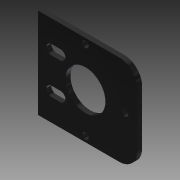
# Autodesk Inventor part: 30288-01
Saved by Autodesk Inventor 2014 (Build 180170000, 170)
## iProperties
Category: NS
Created: 2013-07-17
Part Number: 30288-01
Material: Steel, Mild
Document SubType Name: Modeling
Designer: Edward
Density: 7.86 g/cm^3
Appearance: Lacquer - Black
Description: z-axis motor mount plate (12ga)
Project: Shapeoko
User Status: F
Vendor: ProkTech
Stock Number: SMZM-01
Authority: PER BARRY PROCK 9-16-13 - QUOTE FOR S2ZM-01
Author: Edward
Subject: Structural
Comments: Fusion
Autodesk Inventor part; units mm, degrees
ref_plane "YZ Plane" through (0, 0, 0) normal (1, 0, 0) x (0, 1, 0)
ref_plane "XZ Plane" through (0, 0, 0) normal (0, 1, 0) x (-1, 0, 0)
ref_plane "XY Plane" through (0, 0, 0) normal (0, 0, 1) x (1, 0, 0)
sketch "Sketch1" plane through (0, 0, 0) normal (0, 0, 1) x (1, 0, 0)
  line L0 (-10, -25) -> (45, -25)
  line L1 (45, -25) -> (45, 25)
  line L2 (45, 25) -> (-10, 25)
  line L3 (-10, 25) -> (-10, -25)
  circle A0 centre (16.35, 0) radius 11
  circle A1 centre (38.2703, 0) radius 1.75
  circle A2 centre (16.35, 21.9203) radius 1.75
  circle A3 centre (-5.5703, 0) radius 1.75
  circle A4 centre (16.35, -21.9203) radius 1.75
  line L4 (-2.5, -10) -> (2.5, -10) construction
  line L5 (-2.5, -12.75) -> (2.5, -12.75)
  line L6 (2.5, -7.25) -> (-2.5, -7.25)
  arc A5 (-2.5, -7.25) -> (-2.5, -12.75) centre (-2.5, -10) ccw
  arc A6 (2.5, -12.75) -> (2.5, -7.25) centre (2.5, -10) ccw
  line L7 (-2.5, 7.25) -> (2.5, 7.25)
  line L8 (2.5, 12.75) -> (-2.5, 12.75)
  arc A7 (-2.5, 12.75) -> (-2.5, 7.25) centre (-2.5, 10) ccw
  arc A8 (2.5, 7.25) -> (2.5, 12.75) centre (2.5, 10) ccw
  point P0 (0, 0)
  point P1 (45, 25)
  point P2 (-10, 25)
  point P3 (45, 25)
  point P4 (0, -10)
  dimension "d15" = 0
  dimension "d1" = 22
  dimension "d2" = 25
  dimension "d3" = 26.35
  dimension "d4" = 55
  dimension "d5" = 25
  dimension "d6" = 3.5
  dimension "d7" = 21.9203
  dimension "d8" = 0
  dimension "d11" = 360
  dimension "d13" = 50
  dimension "d14" = 10
  dimension "d16" = 5
  dimension "d17" = 5.5
  dimension "d18" = 10
  dimension "d19" = 15
  dimension "d22" = 20
  constraints: 20 end point, 9 centre point, 8 point on circle, 6 point on line, 5 horizontal, 5 vertical, 4 parallel, 4 tangent, 1 midpoint, 1 perpendicular, 35 other
  measures "d1" diameter of A0
  measures "d2" distance from line of L0 A0.centre
  measures "d3" distance from line of L3 A0.centre
  measures "d4" distance of point (45, 25) point (-10, 25)
  measures "d5" distance from line of point (0, 0) L0
  measures "d6" diameter of A1
  measures "d7" distance of A1.centre A0.centre
  measures "d8" vertical distance of A1.centre A0.centre
  measures "d13" distance of point (45, -25) point (45, 25)
  measures "d14" distance from line of L3 point (0, 0)
  measures "d16" distance of L4.start L4.end
  measures "d17" diameter of A6
  measures "d18" distance from line of L3 point (0, -10)
  measures "d19" distance from line of L0 point (0, -10)
  measures "d22" distance of L6.start L8.start
extrude "Extrusion1" add sketch "Sketch1" along normal blind 2.6568 contours L3 L2 L1 L0 | A3
fillet "Fillet1" radius 10 2 edges at (45, 25, 1.3284) (45, -25, 1.3284)
equation "\"d2\" = d5"
equation "\"d5\" = 0.5 * d13"
body "Solid1"
